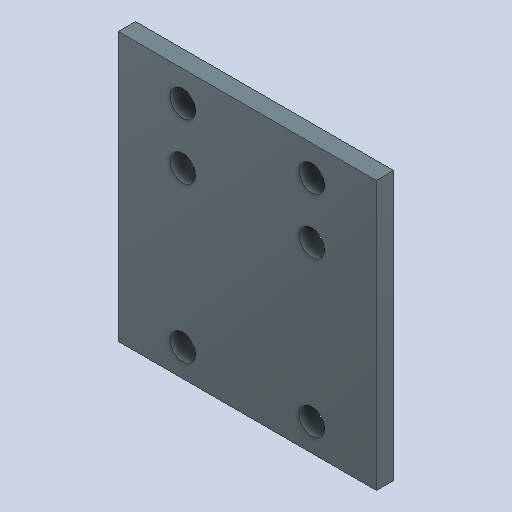
# Autodesk Inventor part: lead_3
Saved by Autodesk Inventor 2023 (Build 270158000, 158)
## iProperties
Created: 2022-12-26
Part Number: lead_3
Material: Lead
Document SubType Name: Modeling
Designer: Kamil
Mass: 28.4314 g
Surface Area: 29.1307 cm^2
Volume: 2.50718 cm^3
Density: 11.34 g/cm^3
Appearance: Lead
Author: Kamil
Autodesk Inventor part; units mm, degrees
ref_plane "YZ Plane" through (0, 0, 0) normal (1, 0, 0) x (0, 1, 0)
ref_plane "XZ Plane" through (0, 0, 0) normal (0, 1, 0) x (-1, 0, 0)
ref_plane "XY Plane" through (0, 0, 0) normal (0, 0, 1) x (1, 0, 0)
sketch "Sketch1" plane through (0, 0, 0) normal (0, 0, 1) x (1, 0, 0)
  line L0 (5.75, -21.6) -> (5.75, 21.6) projected
  line L1 (5.75, 21.6) -> (-5.75, 21.6) projected
  line L2 (-5.75, 21.6) -> (-5.75, -21.6) projected
  line L3 (-5.75, -21.6) -> (5.75, -21.6) projected
  circle A0 centre (-1.75, -18.4) radius 1.5 projected
  circle A1 centre (-1.75, 17.6) radius 1.5 projected
  circle A2 centre (-1.75, -0.4) radius 1.5 projected
  line L4 (-12.75, -21.6) -> (-12.75, 21.6) projected
  line L5 (-12.75, 21.6) -> (-24.25, 21.6) projected
  line L6 (-24.25, 21.6) -> (-24.25, -21.6) projected
  line L7 (-24.25, -21.6) -> (-12.75, -21.6) projected
  circle A3 centre (-16.75, 17.6) radius 1.5 projected
  circle A4 centre (-16.75, -0.4) radius 1.5 projected
  circle A5 centre (-16.75, -18.4) radius 1.5 projected
  line L8 (5.75, -21.6) -> (-24.25, -21.6)
  line L9 (-24.25, -21.6) -> (-24.25, 21.6)
  line L10 (-24.25, 21.6) -> (5.75, 21.6)
  line L11 (5.75, 21.6) -> (5.75, -21.6)
  point P0 (0, 0)
  constraints: 8 end point, 2 parallel, 1 horizontal, 1 perpendicular
extrude "Extrusion1" add sketch "Sketch1" along normal blind 2
sketch "Sketch2" plane through (0, 0, 0) normal (0, 0, -1) x (-1, 0, 0)
  line L0 (-5.75, -21.6) -> (-5.75, 21.6) projected
  line L1 (24.25, -21.6) -> (-5.75, -21.6) projected
  line L2 (24.25, 21.6) -> (24.25, -21.6) projected
  line L3 (-5.75, 21.6) -> (24.25, 21.6) projected
  circle A0 centre (16.75, -18.4) radius 1.5 projected
  circle A1 centre (16.75, -0.4) radius 1.5 projected
  circle A2 centre (16.75, 17.6) radius 1.5 projected
  circle A3 centre (1.75, -0.4) radius 1.5 projected
  circle A4 centre (1.75, 17.6) radius 1.5 projected
  circle A5 centre (1.75, -18.4) radius 1.5 projected
  line L4 (5.2, 10.6) -> (5.2, -18.6)
  line L5 (-5.75, 10.6) -> (5.2, 10.6)
  line L6 (-5.75, -21.6) -> (-5.75, 21.6) projected
  line L7 (24.25, -18.6) -> (24.25, 10.6)
  line L8 (13.3, -18.6) -> (13.3, 10.6)
  line L9 (5.2, -18.6) -> (5.2, -21.6)
  line L10 (13.3, -21.6) -> (13.3, -18.6)
  line L11 (13.3, 10.6) -> (24.25, 10.6)
  line L12 (-5.75, 10.6) -> (5.2, 10.6)
  circle A6 centre (1.75, -0.4) radius 1.75
  circle A7 centre (1.75, 6.1) radius 1.5
  circle A8 centre (16.75, 6.1) radius 1.5
  circle A9 centre (16.75, -0.4) radius 1.75
  point P0 (0, 0)
  point P1 (18.2695, -1.2681)
  constraints: 16 end point, 5 vertical, 3 centre point, 3 horizontal, 19 other
extrude "Extrusion2" cut sketch "Sketch2" against normal blind 10 contours L0 L3 L2 L11 L8 L10 L1 L9 L4 L5 | A7 | A8
sketch "Sketch3" plane through (0, 0, 0) normal (0, 0, -1) x (-1, 0, 0)
  line L0 (5.2, -21.6) -> (-5.75, -21.6) projected
  line L1 (13.3, 10.6) -> (24.25, 10.6)
  line L2 (24.25, -9.4) -> (24.25, 8.7)
  line L3 (24.25, -18.6) -> (24.25, 10.6)
  line L4 (-5.75, -21.6) -> (-5.75, 10.6) projected
  line L5 (24.25, 10.6) -> (24.25, -21.6) projected
  line L6 (24.25, 10.6) -> (-5.75, 10.6)
  line L7 (-5.75, 10.6) -> (-5.75, -21.6)
  line L8 (-5.75, -21.6) -> (24.25, -21.6)
  line L9 (24.25, -21.6) -> (24.25, 10.6)
  line L10 (5.2, -21.6) -> (5.2, 10.6) projected
  line L11 (13.3, 10.6) -> (13.3, -21.6) projected
  point P0 (0, 0)
  constraints: 14 end point, 2 horizontal, 2 parallel, 2 vertical, 1 perpendicular, 5 other
extrude "Extrusion3" add sketch "Sketch3" against normal blind 2 contours L10 L6 L11 L8
sketch "Sketch4" plane through (0, 0, 0) normal (0, 0, -1) x (-1, 0, 0)
  circle A0 centre (1.75, -18.4) radius 1.5 projected
  circle A1 centre (1.75, -0.4) radius 1.5 projected
  circle A2 centre (1.75, 6.1) radius 1.5 projected
  line L0 (24.25, -21.6) -> (-5.75, -21.6) projected
  line L1 (24.25, 10.6) -> (24.25, -21.6) projected
  line L2 (24.25, 10.6) -> (-5.75, 10.6) projected
  line L3 (-5.75, -21.6) -> (-5.75, 10.6) projected
  circle A3 centre (16.75, 6.1) radius 1.5 projected
  circle A4 centre (16.75, -18.4) radius 1.5 projected
  circle A5 centre (16.75, -0.4) radius 1.5 projected
  line L4 (-5.75, 10.6) -> (24.25, 10.6) projected
  line L5 (-5.75, -21.6) -> (-5.75, 10.6) projected
  line L6 (24.25, 10.6) -> (-5.75, 10.6)
  line L7 (-5.75, 10.6) -> (-5.75, 9.6)
  line L8 (-5.75, 9.6) -> (24.25, 9.6)
  line L9 (24.25, 9.6) -> (24.25, 10.6)
  point P0 (0, 0)
  dimension "d6" = 1
  constraints: 8 end point, 2 parallel, 1 horizontal, 1 perpendicular, 1 point on line
  measures "d6" distance of L7.end L6.end
extrude "Extrusion4" cut sketch "Sketch4" against normal blind 2 contours L8 L3 L2 L1
body "Solid1"
